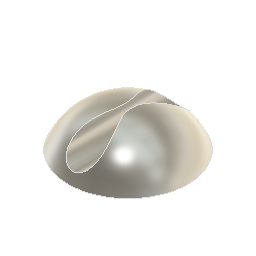
Круглое одинарное крепление проводов (Autodesk Fusion 360 design; units mm, degrees)
Autodesk Fusion 360 part; units mm, degrees
sketch "Sketch1" plane through (0, 0, 0) normal (0, 0, 1) x (1, 0, 0)
  circle A0 centre (0, 0) radius 12.5
  dimension "d1" = 25
  constraint coincident A0.centre origin
  measures "d1" diameter of A0
extrude "Extrude1" add sketch "Sketch1" along normal blind 8
fillet "Fillet1" radius 12.5 1 edges at (-11.6541, -4.5202, 8)
sketch "Sketch2" plane through (0, 0, 0) normal (0, 1, 0) x (1, 0, 0)
  circle A0 centre (0, -5) radius 3.1
  dimension "d6" = 6.2
  measures "d6" diameter of A0
extrude "Extrude2" cut sketch "Sketch2" along normal mid plane 29
